Autodesk Inventor part; units mm, degrees
(part 2 of 2)
  line L391 (45.4044, -128.3159) -> (45.4044, -129.0865)
  line L392 (45.4044, -129.0865) -> (46.7036, -129.0865)
  line L393 (46.7036, -129.0865) -> (46.7036, -129.667)
  line L394 (46.7036, -129.667) -> (44.6436, -129.667)
  dimension "d21" = 2.54
  dimension "d22" = 2.54
  dimension "d23" = 2.54
  dimension "d24" = 5.08
  constraints: 12 tangent, 6 collinear, 5 equal length, 3 centre point, 12 other
  measures "d21" radial gap between concentric circles of A0 A5
  measures "d22" radial gap between concentric circles of A3 A6
  measures "d23" radial gap between concentric circles of A2 A7
  measures "d24" distance of L0.end L1.end
extrude "Extrusion3" cut sketch "Sketch4" against normal blind 1.27
sketch "Sketch5" plane through (0, 0, 0) normal (0, -1, 0) x (1, 0, 0)
  circle A0 centre (21.1667, -76.835) radius 1.5875 projected
  line L0 (72.8133, -76.835) -> (85.5133, -76.835) construction
  circle A1 centre (85.5133, -33.782) radius 1.5875 construction
  circle A2 centre (85.5133, -119.888) radius 1.5875 construction
  line L1 (85.5133, -33.782) -> (85.5133, -119.888) construction
  point P0 (0, 0)
  dimension "d27" = 12.7
  constraints: 4 end point, 1 horizontal, 1 midpoint, 1 point on line, 1 vertical
  measures "d27" distance of L0.start L0.end
hole "Hole2" at (72.8133, 0, -76.835) at (85.5133, 0, -76.835) direction (0, 1, 0) diameter 2.54 end through all counterbore diameter 6.35 counterbore depth 3.175
chamfer "Chamfer1" distance 1.27 angle 45 4 edges at (53.34, 0, 0) (0, 0, -76.835) (106.68, 0, -76.835) (53.34, 0, -153.67)
fillet "Fillet1" radius 3.175 4 edges at (0, 2.2225, -153.67) (0, 2.2225, 0) (106.68, 2.2225, 0) (106.68, 2.2225, -153.67)
equation "\"d8\" = d7"
equation "\"d10\" = d9"
equation "\"d11\" = d10"
equation "\"d12\" = 3 * d10"
equation "\"d13\" = 3 * d7"
equation "\"d22\" = d21"
equation "\"d23\" = d22"
body "Solid1"
